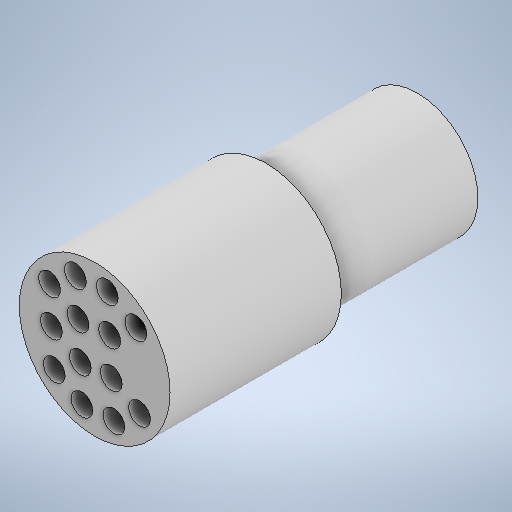
# Autodesk Inventor part: SubConnectorFemale
Saved by Autodesk Inventor 2025.1 (Build 291241020, 241B)
## iProperties
Created: 2025-12-10
Part Number: SubConnectorFemale
Material: Generic
Document SubType Name: Modeling
Designer: tapen
Density: 1 g/cm^3
Appearance: Default
Author: tapen
Autodesk Inventor part; units mm, degrees
ref_plane "YZ Plane" through (0, 0, 0) normal (1, 0, 0) x (0, 1, 0)
ref_plane "XZ Plane" through (0, 0, 0) normal (0, 1, 0) x (-1, 0, 0)
ref_plane "XY Plane" through (0, 0, 0) normal (0, 0, 1) x (1, 0, 0)
sketch "Sketch1" plane through (0, 0, 0) normal (0, 0, 1) x (1, 0, 0)
  line L0 (-32.804, 25.0779) -> (43.5584, 25.0779) construction
  line L1 (43.5584, 25.0779) -> (43.5584, -32.1939) construction
  line L2 (43.5584, -32.1939) -> (-32.804, -32.1939) construction
  line L3 (-32.804, -32.1939) -> (-32.804, 25.0779) construction
  circle A0 centre (0, 0) radius 12.45
  circle A1 centre (-2.7452, 2.9307) radius 1.8
  circle A2 centre (2.0802, 9.2435) radius 1.8
  circle A3 centre (6.8191, 6.4677) radius 1.8
  circle A4 centre (2.4803, 3.2418) radius 1.8
  circle A5 centre (2.7429, -2.735) radius 1.8
  circle A6 centre (7.4192, -5.4857) radius 1.8
  circle A7 centre (3.168, -8.6867) radius 1.8
  circle A8 centre (-2.121, -8.9618) radius 1.8
  circle A9 centre (-6.6849, -6.261) radius 1.8
  circle A10 centre (-2.3836, -3.06) radius 1.8
  circle A11 centre (-7.1475, -0.2717) radius 1.8
  circle A12 centre (-7.4476, 5.6175) radius 1.8
  circle A13 centre (-3.1838, 8.9184) radius 1.8
  point P0 (1.2025, 0.5328)
  point P1 (1.2025, 0.5328)
  point P2 (10.2924, 3.877)
  point P3 (10.2924, 3.877)
  point P4 (7.8667, 0.451)
  point P5 (7.8667, 0.451)
  point P6 (8.992, -0.5743)
  point P7 (8.992, -0.5743)
  point P8 (9.5046, -4.6505)
  point P9 (9.5046, -4.6505)
  point P10 (6.5538, -10.4772)
  point P11 (6.5538, -10.4772)
  point P12 (1.8524, -12.6278)
  point P13 (1.8524, -12.6278)
  point P14 (-4.637, -8.6017)
  point P15 (-4.637, -8.6017)
  point P16 (1.3898, -6.9012)
  point P17 (1.3898, -6.9012)
  point P18 (-4.7995, -2.8875)
  point P19 (-4.7995, -2.8875)
  point P20 (-5.0121, 2.6391)
  point P21 (-5.0121, 2.6391)
  point P22 (0.502, 5.665)
  point P23 (0.502, 5.665)
  dimension "d3" = 24.9
  dimension "d99" = 3.6
  dimension "d100" = 3.6
  dimension "d101" = 3.6
  dimension "d102" = 3.6
  dimension "d103" = 3.6
  dimension "d104" = 3.6
  dimension "d105" = 3.6
  dimension "d106" = 3.6
  dimension "d107" = 3.6
  dimension "d108" = 3.6
  dimension "d109" = 3.6
  dimension "d110" = 3.6
  dimension "d111" = 3.6
  constraints: 14 centre point, 13 coincident, 2 other
  measures "d3" diameter of A0
  measures "d99" diameter of A10
  measures "d100" diameter of A1
  measures "d101" diameter of A13
  measures "d102" diameter of A12
  measures "d103" diameter of A11
  measures "d104" diameter of A9
  measures "d105" diameter of A8
  measures "d106" diameter of A7
  measures "d107" diameter of A6
  measures "d108" diameter of A5
  measures "d109" diameter of A4
  measures "d110" diameter of A3
  measures "d111" diameter of A2
extrude "Extrusion1" add sketch "Sketch1" along normal blind 17
sketch "Sketch2" plane through (0, 0, 0) normal (0, 0, -1) x (-1, 0, 0)
  circle A0 centre (0, 0) radius 12.45
  constraints: 1 centre point, 1 coincident
extrude "Extrusion2" add sketch "Sketch2" along normal blind 11.3
sketch "Sketch3" plane through (0, 0, -11.3) normal (0, 0, -1) x (-1, 0, 0)
  circle A0 centre (0, 0) radius 10
  dimension "d96" = 20
  constraints: 1 centre point, 1 coincident
  measures "d96" diameter of A0
extrude "Extrusion3" add sketch "Sketch3" along normal blind 25
equation "\"d100\" = d99"
equation "\"d101\" = d99"
equation "\"d102\" = d99"
equation "\"d103\" = d99"
equation "\"d104\" = d99"
equation "\"d105\" = d99"
equation "\"d106\" = d99"
equation "\"d107\" = d99"
equation "\"d108\" = d99"
equation "\"d109\" = d99"
equation "\"d110\" = d99"
equation "\"d111\" = d99"
body "Solid1"
